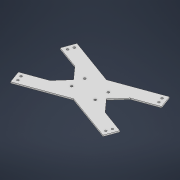
# Autodesk Inventor part: Kreuz_Halterung
Saved by Autodesk Inventor 2021 (Build 250183000, 183)
## iProperties
Created: 2021-02-01
Part Number: Kreuz_Halterung
Material: Generisch
Document SubType Name: Modeling
Designer: laure
Density: 1 g/cm^3
Appearance: Vorgabe
Author: laure
Autodesk Inventor part; units mm, degrees
ref_plane "YZ Plane" through (0, 0, 0) normal (1, 0, 0) x (0, 1, 0)
ref_plane "XZ Plane" through (0, 0, 0) normal (0, 1, 0) x (-1, 0, 0)
ref_plane "XY Plane" through (0, 0, 0) normal (0, 0, 1) x (1, 0, 0)
sketch "Skizze1" plane through (0, 0, 0) normal (0, 1, 0) x (-1, 0, 0)
  line L0 (25, -25) -> (-25, -25)
  line L1 (-25, -25) -> (-25, 25)
  line L2 (-25, 25) -> (25, 25)
  line L3 (25, 25) -> (25, -25)
  line L4 (0, -70.9121) -> (0, 70.9121) projected
  line L5 (0, -25) -> (-70.4769, -50.6515)
  line L6 (-70.4769, -50.6515) -> (-77.3173, -31.8577)
  line L7 (-77.3173, -31.8577) -> (-42.0428, -19.0188)
  line L8 (575.1827, 0) -> (-605.81, 0) projected
  line L9 (0, -25) -> (70.4769, -50.6515)
  line L10 (70.4769, -50.6515) -> (77.3173, -31.8577)
  line L11 (77.3173, -31.8577) -> (42.0428, -19.0188)
  line L12 (-575.1827, 0) -> (605.81, 0)
  line L13 (0, 25) -> (-70.4769, 50.6515)
  line L14 (-70.4769, 50.6515) -> (-77.3173, 31.8577)
  line L15 (-77.3173, 31.8577) -> (-42.0428, 19.0188)
  line L16 (77.3173, 31.8577) -> (42.0428, 19.0188)
  line L17 (0, 25) -> (70.4769, 50.6515)
  line L18 (70.4769, 50.6515) -> (77.3173, 31.8577)
  line L19 (-42.0428, -19.0188) -> (-25, 0)
  line L20 (42.0428, -19.0188) -> (25, 0)
  line L21 (-42.0428, 19.0188) -> (-25, 0)
  line L22 (42.0428, 19.0188) -> (25, 0)
  point P0 (0, 0)
  dimension "d0" = 50
  dimension "d1" = 50
  dimension "d3" = 75
  dimension "d6" = 20
  dimension "d7" = 20
  dimension "d8" = 90
  dimension "d12" = 41.864
  constraints: 42 end point, 13 symmetric about line, 2 midpoint, 2 parallel, 2 perpendicular, 2 point on line, 1 horizontal, 2 other
  measures "d0" distance of L1.end L2.end
  measures "d1" distance of L0.end L1.end
  measures "d3" distance of L5.start L5.end
  measures "d6" angle of L0 L5
  measures "d7" distance of L5.end L6.end
  measures "d8" angle of L6 L5
  measures "d12" angle of L1 L19
extrude "Extrusion1" add sketch "Skizze1" along normal blind 2
sketch "Skizze2" plane through (0, 2, 0) normal (0, 1, 0) x (1, 0, 0)
  circle A0 centre (-66.8909, 42.9612) radius 1.6
  line L0 (0, 25) -> (-70.4769, 50.6515) projected
  line L1 (-70.4769, 50.6515) -> (-77.3173, 31.8577) projected
  circle A1 centre (-69.6271, 35.4437) radius 1.6
  line L2 (-77.3173, 31.8577) -> (-42.0428, 19.0188) projected
  line L3 (0, 79.2706) -> (0, -73.1803) projected
  line L4 (127.2474, 0) -> (-133.3376, 0) projected
  circle A2 centre (66.8909, 42.9612) radius 1.6
  circle A3 centre (69.6271, 35.4437) radius 1.6
  circle A4 centre (-66.8909, -42.9612) radius 1.6
  circle A5 centre (-69.6271, -35.4437) radius 1.6
  circle A6 centre (66.8909, -42.9612) radius 1.6
  circle A7 centre (69.6271, -35.4437) radius 1.6
  point P0 (0, 0)
  dimension "d15" = 3.2
  dimension "d16" = 6
  dimension "d17" = 6
  dimension "d18" = 3.2
  dimension "d19" = 6
  dimension "d20" = 6
  constraints: 8 centre point, 6 symmetric about line, 6 other
  measures "d15" diameter of A0
  measures "d16" distance from line of A0.centre L0
  measures "d17" distance from line of L1 A0.centre
  measures "d18" diameter of A1
  measures "d19" distance from line of A1.centre L2
  measures "d20" distance from line of L1 A1.centre
extrude "Extrusion2" cut sketch "Skizze2" against normal up to surface (2 mm away)
sketch "Skizze3" plane through (0, 2, 0) normal (0, 1, 0) x (1, 0, 0)
  circle A0 centre (-18, 10) radius 1.6
  line L0 (0, 70.9121) -> (0, -70.9121) projected
  line L1 (108.2443, 0) -> (-108.2443, 0) projected
  circle A1 centre (-18, -10) radius 1.6
  circle A2 centre (18, 10) radius 1.6
  circle A3 centre (18, -10) radius 1.6
  point P0 (0, 0)
  dimension "d23" = 3.2
  dimension "d24" = 18
  dimension "d25" = 10
  constraints: 4 centre point, 3 symmetric about line, 3 other
  measures "d23" diameter of A0
  measures "d24" distance from line of L0 A0.centre
  measures "d25" distance from line of L1 A0.centre
extrude "Extrusion3" cut sketch "Skizze3" against normal up to surface (2 mm away)
